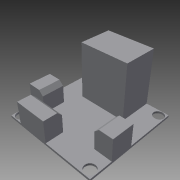
# Autodesk Inventor part: Motor Shield l298
Saved by Autodesk Inventor 2015 (Build 190159000, 159)
## iProperties
Created: 2019-01-15
Part Number: Motor Shield l298
Material: Типовые
Document SubType Name: Modeling
Designer: kostya
Density: 1 g/cm^3
Appearance: По умолчанию
Author: kostya
Autodesk Inventor part; units mm, degrees
ref_plane "YZ Plane" through (0, 0, 0) normal (1, 0, 0) x (0, 1, 0)
ref_plane "XZ Plane" through (0, 0, 0) normal (0, 1, 0) x (-1, 0, 0)
ref_plane "XY Plane" through (0, 0, 0) normal (0, 0, 1) x (1, 0, 0)
sketch "Эскиз1" plane through (0, 0, 0) normal (0, 0, 1) x (1, 0, 0)
  line L0 (-21.5, -21.5) -> (21.5, -21.5)
  line L1 (21.5, -21.5) -> (21.5, 21.5)
  line L2 (21.5, 21.5) -> (-21.5, 21.5)
  line L3 (-21.5, 21.5) -> (-21.5, -21.5)
  line L4 (-21.5, -21.5) -> (21.5, 21.5) construction
  line L5 (21.5, -21.5) -> (-21.5, 21.5) construction
  line L6 (-21.5, 21.5) -> (-20.5, 21.5) construction
  line L7 (-20.5, 21.5) -> (-20.5, 20.5) construction
  line L8 (-20.5, 20.5) -> (-16.9645, 16.9645) construction
  circle A0 centre (-18.7322, 18.7322) radius 2.5
  line L9 (0, 21.5) -> (0, -21.5) construction
  line L10 (-21.5, 0) -> (21.5, 0) construction
  circle A1 centre (18.7322, 18.7322) radius 2.5
  line L11 (21.5, 0) -> (-21.5, 0) construction
  circle A2 centre (-18.7322, -18.7322) radius 2.5
  circle A3 centre (18.7322, -18.7322) radius 2.5
  point P0 (0, 0)
  dimension "d0" = 43
  dimension "d1" = 43
  dimension "d2" = 1
  dimension "d3" = 1
  dimension "d4" = 5
  constraints: 24 end point, 7 midpoint, 5 symmetric about line, 3 centre point, 3 point on line, 2 parallel, 1 horizontal, 1 perpendicular, 6 other
  measures "d0" distance of L2.end L1.end
  measures "d1" distance of L1.end L0.end
  measures "d2" distance of L2.end L6.end
  measures "d3" distance of L6.end L7.end
  measures "d4" distance of L7.end L8.end
extrude "Выдавливание1" add sketch "Эскиз1" along normal blind 1
sketch "Эскиз2" plane through (0, 0, 1) normal (0, 0, 1) x (1, 0, 0)
  circle A0 centre (18.7322, -18.7322) radius 2.5 projected
  circle A1 centre (-18.7322, -18.7322) radius 2.5 projected
  circle A2 centre (18.7322, 18.7322) radius 2.5 projected
  circle A3 centre (-18.7322, 18.7322) radius 2.5 projected
  line L0 (-21.5, -21.5) -> (21.5, -21.5) projected
  line L1 (21.5, -21.5) -> (21.5, 21.5) projected
  line L2 (21.5, 21.5) -> (-21.5, 21.5) projected
  line L3 (-21.5, 21.5) -> (-21.5, -21.5) projected
  line L4 (21.5, 21.5) -> (-21.5, 21.5) construction
  line L5 (0, 21.5) -> (0, 0) construction
  line L6 (0, 21.5) -> (11, 21.5)
  line L7 (0, 21.5) -> (-11, 21.5)
  line L8 (-11, 21.5) -> (11, 21.5)
  line L9 (11, 21.5) -> (11, 6.5)
  line L10 (11, 6.5) -> (-11, 6.5)
  line L11 (-11, 6.5) -> (-11, 21.5)
  dimension "d7" = 11
  dimension "d8" = 11
  dimension "d9" = 15
  constraints: 14 end point, 2 parallel, 2 point on line, 1 horizontal, 1 midpoint, 1 perpendicular, 1 vertical
  measures "d7" distance of L5.start L6.end
  measures "d8" distance of L5.start L7.end
  measures "d9" distance of L8.end L9.end
extrude "Выдавливание2" add sketch "Эскиз2" along normal blind 25 contours L2 L9 L10 L11
sketch "Эскиз3" plane through (0, 0, 1) normal (0, 0, 1) x (1, 0, 0)
  line L0 (-11, 6.5) -> (-11, 21.5) projected
  line L1 (-11, 21.5) -> (-21.5, 21.5) projected
  line L2 (-21.5, 21.5) -> (-21.5, -21.5) projected
  line L3 (-21.5, -21.5) -> (21.5, -21.5) projected
  line L4 (21.5, -21.5) -> (21.5, 21.5) projected
  line L5 (21.5, 21.5) -> (11, 21.5) projected
  line L6 (11, 21.5) -> (11, 6.5) projected
  line L7 (11, 6.5) -> (-11, 6.5) projected
  circle A0 centre (18.7322, -18.7322) radius 2.5 projected
  circle A1 centre (-18.7322, -18.7322) radius 2.5 projected
  circle A2 centre (18.7322, 18.7322) radius 2.5 projected
  circle A3 centre (-18.7322, 18.7322) radius 2.5 projected
  line L8 (-21.5, 21.5) -> (-21.5, -1.5) construction
  line L9 (-21.5, 21.5) -> (-21.5, -21.5) projected
  line L10 (-21.5, -1.5) -> (-13.5, -1.5)
  line L11 (-13.5, -1.5) -> (-13.5, -11.5)
  line L12 (-13.5, -11.5) -> (-21.5, -11.5)
  line L13 (-21.5, -11.5) -> (-21.5, -1.5) construction
  line L14 (-21.5, -1.5) -> (-21.5, -11.5)
  line L15 (-16.2322, -18.7322) -> (-15.2322, -18.7322) construction
  line L16 (-15.2322, -18.7322) -> (-15.2322, -15.4295) construction
  line L17 (-15.2322, -18.7322) -> (-15.2322, -21.5) construction
  line L18 (-15.2322, -21.5) -> (-0.2322, -21.5)
  line L19 (-0.2322, -21.5) -> (-0.2322, -13.5)
  line L20 (-0.2322, -13.5) -> (-15.2322, -13.5)
  line L21 (-15.2322, -13.5) -> (-15.2322, -21.5)
  point P0 (0, 0)
  dimension "d21" = 2
  dimension "d13" = 23
  dimension "d14" = 8
  dimension "d15" = 10
  dimension "d16" = 1
  dimension "d17" = 15
  dimension "d18" = 8
  constraints: 26 end point, 4 parallel, 4 perpendicular, 3 horizontal, 2 point on line, 1 collinear, 1 horizontal alignment, 1 other
  measures "d13" distance of L1.end L8.end
  measures "d14" distance of L11.end L12.end
  measures "d15" distance of L10.end L11.end
  measures "d16" distance of L15.start L15.end
  measures "d17" distance of L20.end L19.end
  measures "d18" distance of L19.end L18.end
extrude "Выдавливание3" add sketch "Эскиз3" along normal blind 10 contours L3 L21 L20 L19
ref_plane "РабПлоскость1" through (0, -21.5, 0) normal (1, 0, 0) x (0, 0, -1)
extrude "Выдавливание4" add sketch "Эскиз3" along normal blind 10 contours L10 L11 L12 L2
mirror "Зеркальное отражение1" about plane through (0, -21.5, 0) normal (1, 0, 0) of "Выдавливание4"
chamfer "Фаска1" distance 2 angle 45 3 edges at (-7.7322, -13.5, 11) (-13.5, -6.5, 11) (13.5, -6.5, 11)
